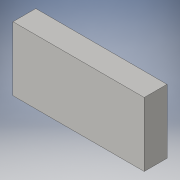
# Autodesk Inventor part: mcdave_battery
Saved by Autodesk Inventor 2016 (Build 200138000, 138)
## iProperties
Created: 2017-08-31
Part Number: mcdave_battery
Material: Generic
Document SubType Name: Modeling
Designer: student
Density: 1 g/cm^3
Appearance: Default
Author: student
Autodesk Inventor part; units mm, degrees
ref_plane "YZ Plane" through (0, 0, 0) normal (1, 0, 0) x (0, 1, 0)
ref_plane "XZ Plane" through (0, 0, 0) normal (0, 1, 0) x (-1, 0, 0)
ref_plane "XY Plane" through (0, 0, 0) normal (0, 0, 1) x (1, 0, 0)
sketch "Sketch1" plane through (0, 0, 0) normal (0, 0, 1) x (1, 0, 0)
  line L0 (-28.1651, 13.0672) -> (41.1261, 13.0672)
  line L1 (41.1261, 13.0672) -> (41.1261, -20.7656)
  line L2 (41.1261, -20.7656) -> (-28.1651, -20.7656)
  line L3 (-28.1651, -20.7656) -> (-28.1651, 13.0672)
  point P0 (0, 0)
  dimension "d0" = 33.8328
  dimension "d1" = 69.2912
  constraints: 8 end point, 2 parallel, 1 horizontal, 1 perpendicular
  measures "d0" distance of L0.end L1.end
  measures "d1" distance of L0.start L0.end
extrude "Extrusion1" add sketch "Sketch1" along normal blind 12.0396
body "Solid1"
